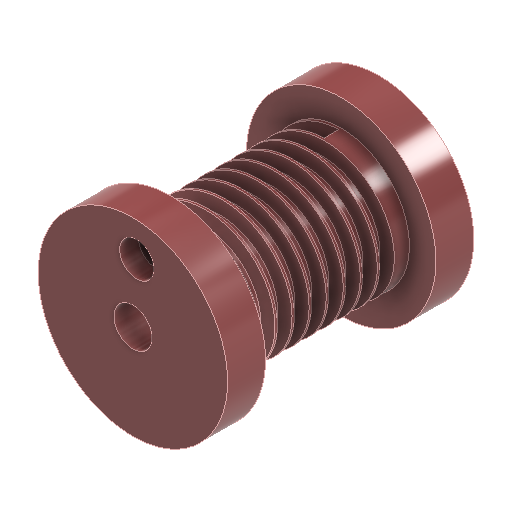
# Autodesk Inventor part: carrete
Saved by Autodesk Inventor 2026.1 (Build 301233000, 233)
## iProperties
Created: 2025-06-24
Part Number: carrete
Material: Genérico
Document SubType Name: Modeling
Designer: piero
Density: 1 g/cm^3
Appearance: Castaño
Author: piero
Autodesk Inventor part; units mm, degrees
ref_plane "YZ Plane" through (0, 0, 0) normal (1, 0, 0) x (0, 1, 0)
ref_plane "XZ Plane" through (0, 0, 0) normal (0, 1, 0) x (-1, 0, 0)
ref_plane "XY Plane" through (0, 0, 0) normal (0, 0, 1) x (1, 0, 0)
sketch "Boceto1" plane through (0, 0, 0) normal (0, 0, 1) x (1, 0, 0)
  circle A0 centre (0, 0) radius 25
  circle A1 centre (0, 0) radius 4
  circle A2 centre (0, 0) radius 11
  dimension "d0" = 50
  dimension "d3" = 8
  dimension "d34" = 22
  constraints: 3 centre point, 3 coincident
  measures "d0" diameter of A0
  measures "d3" diameter of A1
  measures "d34" diameter of A2
extrude "Extrusión1" add sketch "Boceto1" along normal blind 10 contours A0 | A2
sketch "Boceto5" plane through (0, 0, 10) normal (0, 0, 1) x (1, 0, 0)
  circle A0 centre (0, 0) radius 5
  circle A1 centre (0, 0) radius 18
  dimension "d15" = 10
  dimension "d16" = 36
  constraints: 2 centre point, 2 coincident
  measures "d15" diameter of A0
  measures "d16" diameter of A1
extrude "Extrusión5" add sketch "Boceto5" along normal blind 45
sketch "Boceto6" plane through (0, 0, 55) normal (0, 0, 1) x (1, 0, 0)
  circle A0 centre (0, 0) radius 4 projected
  circle A1 centre (0, 0) radius 25
  circle A2 centre (0, 0) radius 4
  circle A3 centre (0, 0) radius 5 projected
  circle A4 centre (0, 0) radius 11
  dimension "d22" = 50
  dimension "d30" = 8
  dimension "d31" = 22
  constraints: 3 centre point, 2 coincident
  measures "d22" diameter of A1
  measures "d30" diameter of A2
  measures "d31" diameter of A4
extrude "Extrusión6" add sketch "Boceto6" along normal blind 10 contours A1 | A4
sketch "Boceto18" plane through (0, 0, 0) normal (1, 0, 0) x (0, 1, 0)
  line L0 (18, 10) -> (18, 55)
  line L1 (18, 55) -> (18, 51.125446)
  line L2 (18, 10) -> (18, 55)
  line L3 (18, 55) -> (18, 51.125446)
  line L4 (18, 51.125446) -> (15, 51.901299)
  line L5 (15, 51.901299) -> (15, 54.224147)
  line L6 (15, 54.224147) -> (18, 55)
  circle A0 centre (16.5, 53.062723) radius 1.5
  point P0 (0, 0)
  dimension "d109" = 3
  dimension "d110" = 3
  dimension "d127" = 29
  constraints: 11 end point, 3 tangent, 1 centre point, 1 collinear, 1 equal length, 2 other
  measures "d109" distance between parallel lines of L0 L5
  measures "d110" diameter of A0
  measures "d127" angle of L6 L4
coil "Bobina1" sketch "Boceto18" operation cut axis through (0, 0, -10) along (0, 0, -1) pitch 4.5 turns 9 hand right
sketch "Boceto19" plane through (0, 0, 65) normal (0, 0, 1) x (1, 0, 0)
  circle A0 centre (1.75, 16.658331) radius 1.75
  line L0 (0, 15) -> (0, 18)
  circle A1 centre (0, 0) radius 5
  line L1 (0, 18) -> (0, 0) construction
  circle A2 centre (0, 0) radius 15 construction
  dimension "d111" = 3.5
  dimension "d114" = 30
  constraints: 2 centre point, 2 end point, 2 tangent, 1 coincident, 1 vertical
  measures "d111" diameter of A0
  measures "d114" diameter of A2
extrude "Extrusión13" cut sketch "Boceto19" against normal blind 13 contours A0
sketch "Boceto20" plane through (0, 0, 55) normal (0, 0, -1) x (-1, 0, 0)
  arc A0 (0, 15) -> (-1.567164, 14.917909) centre (0, 0) ccw
  arc A1 (0, 18) -> (-0.614031, 17.989524) centre (0, 0) ccw
  line L0 (0, 15) -> (0, 18)
  circle A2 centre (-1.75, 16.658331) radius 1.75
  arc A3 (-1.567164, 14.917909) -> (-0.614031, 17.989524) centre (-1.75, 16.658331) ccw
  point P0 (0, 16.658331)
  point P1 (-1.567164, 14.917909)
  point P2 (-0.614031, 17.989524)
  constraints: 6 point on circle, 3 centre point, 3 coincident, 2 end point, 1 vertical
extrude "Extrusión14" add sketch "Boceto20" along normal blind 4.2 contours A0 A2 L0 | A2 A1 L0
sketch "Boceto24" plane through (0, 0, 65) normal (0, 0, 1) x (1, 0, 0)
  circle A0 centre (1, 16) radius 4.5
  point P0 (0, 0)
  dimension "d128" = 9
  constraints: 1 centre point
  measures "d128" diameter of A0
extrude "Extrusión16" cut sketch "Boceto24" against normal blind 5
